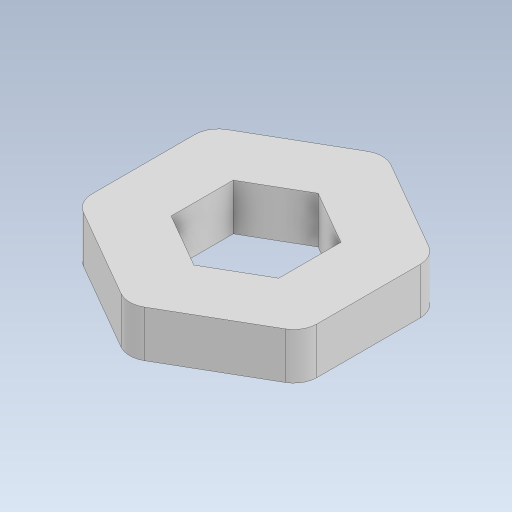
# Autodesk Inventor part: Bolt Head
Saved by Autodesk Inventor 2023 (Build 270158000, 158)
## iProperties
Created: 2022-09-17
Part Number: Bolt Head
Material: Generic
Document SubType Name: Modeling
Designer: Dave
Density: 1 g/cm^3
Appearance: Default
Author: Dave
Autodesk Inventor part; units mm, degrees
ref_plane "YZ Plane" through (0, 0, 0) normal (1, 0, 0) x (0, 1, 0)
ref_plane "XZ Plane" through (0, 0, 0) normal (0, 1, 0) x (-1, 0, 0)
ref_plane "XY Plane" through (0, 0, 0) normal (0, 0, 1) x (1, 0, 0)
sketch "Sketch1" plane through (0, 0, 0) normal (0, 1, 0) x (-1, 0, 0)
  line L0 (7.3612, -4.25) -> (0, -8.5)
  line L1 (0, -8.5) -> (-7.3612, -4.25)
  line L2 (-7.3612, -4.25) -> (-7.3612, 4.25)
  line L3 (-7.3612, 4.25) -> (0, 8.5)
  line L4 (0, 8.5) -> (7.3612, 4.25)
  line L5 (7.3612, 4.25) -> (7.3612, -4.25)
  line L6 (15.3979, -8.89) -> (0, -17.78)
  line L7 (0, -17.78) -> (-15.3979, -8.89)
  line L8 (-15.3979, -8.89) -> (-15.3979, 8.89)
  line L9 (-15.3979, 8.89) -> (0, 17.78)
  line L10 (0, 17.78) -> (15.3979, 8.89)
  line L11 (15.3979, 8.89) -> (15.3979, -8.89)
  point P0 (0, 0)
  point P1 (0, 0)
  point P2 (0, 0)
  dimension "d0" = 8.5
  dimension "d1" = 17.78
  constraints: 24 end point, 2 coincident, 2 vertical, 26 other
  measures "d0" distance of L4.end L0.start
  measures "d1" distance of L10.end L6.start
extrude "Extrusion1" add sketch "Sketch1" along normal blind 6.35
fillet "Fillet1" radius 3.175 6 edges at (-15.3979, 3.175, 8.89) (0, 3.175, 17.78) (15.3979, 3.175, 8.89) (15.3979, 3.175, -8.89) (0, 3.175, -17.78) (-15.3979, 3.175, -8.89)
body "Solid1"
